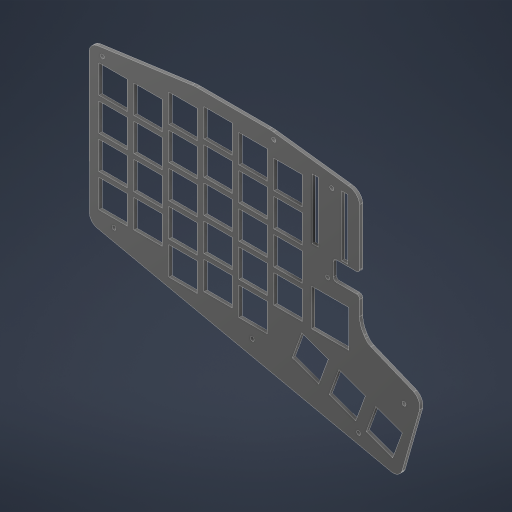
# Autodesk Inventor part: Top plate Right
Saved by Autodesk Inventor 2024.3 (Build 283343000, 343)
## iProperties
Created: 2024-12-13
Part Number: Top plate Right
Material: ABS Plastic
Document SubType Name: Modeling
Designer: micha
Density: 1.06 g/cm^3
Appearance: Smooth - Black
Author: micha
Autodesk Inventor part; units mm, degrees
ref_plane "YZ Plane" through (0, 0, 0) normal (1, 0, 0) x (0, 1, 0)
ref_plane "XZ Plane" through (0, 0, 0) normal (0, 1, 0) x (-1, 0, 0)
ref_plane "Work Plane1" through (0, 0, 0) normal (0, 0, 1) x (1, 0, 0)
sketch "Sketch1" plane through (0, 0, 0) normal (0, 0, 1) x (1, 0, 0)
  arc A0 (218.5045, -64.8588) -> (212.539, -59.4694) centre (212.5401, -65.4644) ccw projected
  line L0 (174.0364, -54.7609) -> (212.539, -59.4694) projected
  arc A1 (174.0364, -54.7609) -> (171.7239, -54.62) centre (171.7239, -73.6702) ccw projected
  line L1 (134.8832, -54.62) -> (171.7239, -54.62) projected
  arc A2 (134.8832, -54.62) -> (132.2802, -54.7987) centre (134.8832, -73.6711) ccw projected
  line L2 (83.5422, -61.5211) -> (132.2802, -54.7987) projected
  arc A3 (83.5422, -61.5211) -> (79.23, -66.4736) centre (84.23, -66.4736) ccw projected
  line L3 (79.4773, -138.0224) -> (79.23, -66.4736) projected
  arc A4 (79.4773, -138.0224) -> (82.9877, -142.7953) centre (84.4773, -138.0223) ccw projected
  line L4 (234.3607, -175.7237) -> (82.9877, -142.7953) projected
  arc A5 (234.3607, -175.7237) -> (240.2338, -172.8773) centre (235.7454, -171.0986) ccw projected
  line L5 (249.3284, -140.9769) -> (240.2338, -172.8773) projected
  arc A6 (249.3284, -140.9769) -> (246.2558, -134.3964) centre (243.557, -139.6641) ccw projected
  line L6 (224.2532, -125.4096) -> (246.2558, -134.3964) projected
  arc A7 (221.4228, -123.1302) -> (224.2532, -125.4096) centre (226.6543, -119.531) ccw projected
  line L7 (220.6818, -122.0531) -> (221.4228, -123.1302) projected
  arc A8 (218.4447, -114.8395) -> (220.6818, -122.0531) centre (231.1445, -114.8548) ccw projected
  line L8 (218.5045, -64.8588) -> (218.4447, -114.8395) projected
  circle A9 centre (163.195, -152.4) radius 1.05 projected
  circle A10 centre (92.075, -138.43) radius 1.05 projected
  circle A11 centre (86.11, -127.04) radius 0.8509 projected
  circle A12 centre (91.61, -127.04) radius 1.7145 projected
  circle A13 centre (97.11, -127.04) radius 0.8509 projected
  circle A14 centre (104.11, -127.04) radius 0.8509 projected
  circle A15 centre (122.11, -139.04) radius 0.8509 projected
  circle A16 centre (122.61, -135.29) radius 1.5 projected
  circle A17 centre (109.61, -127.04) radius 1.7145 projected
  circle A18 centre (115.11, -127.04) radius 0.8509 projected
  circle A19 centre (86.61, -123.29) radius 1.5 projected
  circle A20 centre (91.61, -121.09) radius 1.5 projected
  circle A21 centre (96.61, -123.29) radius 1.5 projected
  circle A22 centre (104.61, -123.29) radius 1.5 projected
  circle A23 centre (109.61, -121.09) radius 1.5 projected
  circle A24 centre (114.61, -123.29) radius 1.5 projected
  circle A25 centre (122.11, -122.04) radius 0.8509 projected
  circle A26 centre (122.61, -118.29) radius 1.5 projected
  circle A27 centre (127.61, -139.04) radius 1.7145 projected
  circle A28 centre (133.11, -139.04) radius 0.8509 projected
  circle A29 centre (132.61, -135.29) radius 1.5 projected
  circle A30 centre (140.11, -136.54) radius 0.8509 projected
  circle A31 centre (127.61, -133.09) radius 1.5 projected
  circle A32 centre (140.61, -132.79) radius 1.5 projected
  circle A33 centre (145.61, -136.54) radius 1.7145 projected
  circle A34 centre (151.11, -136.54) radius 0.8509 projected
  circle A35 centre (158.11, -139.04) radius 0.8509 projected
  circle A36 centre (163.61, -139.04) radius 1.7145 projected
  circle A37 centre (158.61, -135.29) radius 1.5 projected
  circle A38 centre (145.61, -130.59) radius 1.5 projected
  circle A39 centre (150.61, -132.79) radius 1.5 projected
  circle A40 centre (163.61, -133.09) radius 1.5 projected
  circle A41 centre (127.61, -122.04) radius 1.7145 projected
  circle A42 centre (133.11, -122.04) radius 0.8509 projected
  circle A43 centre (140.11, -119.54) radius 0.8509 projected
  circle A44 centre (127.61, -116.09) radius 1.5 projected
  circle A45 centre (132.61, -118.29) radius 1.5 projected
  circle A46 centre (140.61, -115.79) radius 1.5 projected
  circle A47 centre (145.61, -119.54) radius 1.7145 projected
  circle A48 centre (151.11, -119.54) radius 0.8509 projected
  circle A49 centre (158.11, -122.04) radius 0.8509 projected
  circle A50 centre (163.61, -122.04) radius 1.7145 projected
  circle A51 centre (145.61, -113.59) radius 1.5 projected
  circle A52 centre (150.61, -115.79) radius 1.5 projected
  circle A53 centre (158.61, -118.29) radius 1.5 projected
  circle A54 centre (163.61, -116.09) radius 1.5 projected
  circle A55 centre (198.2508, -148.0493) radius 0.8509 projected
  circle A56 centre (187.9141, -144.2871) radius 0.8509 projected
  circle A57 centre (193.0824, -146.1682) radius 1.7145 projected
  circle A58 centre (189.6666, -140.9342) radius 1.5 projected
  circle A59 centre (199.0635, -144.3544) radius 1.5 projected
  circle A60 centre (195.1175, -140.577) radius 1.5 projected
  circle A61 centre (217.8966, -166.9609) radius 1.05 projected
  circle A62 centre (217.2795, -154.9752) radius 0.8509 projected
  circle A63 centre (236.3083, -161.9011) radius 0.8509 projected
  circle A64 centre (225.9717, -158.1389) radius 0.8509 projected
  circle A65 centre (231.14, -160.02) radius 1.7145 projected
  circle A66 centre (227.7241, -154.7861) radius 1.5 projected
  circle A67 centre (237.121, -158.2063) radius 1.5 projected
  circle A68 centre (233.175, -154.4288) radius 1.5 projected
  circle A69 centre (206.9429, -151.213) radius 0.8509 projected
  circle A70 centre (212.1112, -153.0941) radius 1.7145 projected
  circle A71 centre (208.6953, -147.8601) radius 1.5 projected
  circle A72 centre (218.0923, -151.2803) radius 1.5 projected
  circle A73 centre (214.1462, -147.5029) radius 1.5 projected
  circle A74 centre (241.3, -142.24) radius 1.05 projected
  circle A75 centre (169.11, -139.04) radius 0.8509 projected
  circle A76 centre (168.61, -135.29) radius 1.5 projected
  circle A77 centre (201.8629, -128.353) radius 0.8509 projected
  circle A78 centre (169.11, -122.04) radius 0.8509 projected
  circle A79 centre (176.11, -124.54) radius 0.8509 projected
  circle A80 centre (181.61, -124.54) radius 1.7145 projected
  circle A81 centre (176.61, -120.79) radius 1.5 projected
  circle A82 centre (168.61, -118.29) radius 1.5 projected
  circle A83 centre (181.61, -118.59) radius 1.5 projected
  circle A84 centre (187.11, -124.54) radius 0.8509 projected
  circle A85 centre (186.61, -120.79) radius 1.5 projected
  circle A86 centre (194.5006, -125.0592) radius 0.4 projected
  circle A87 centre (194.5006, -123.0592) radius 0.381 projected
  circle A88 centre (194.5006, -121.0592) radius 0.381 projected
  circle A89 centre (201.3506, -114.2092) radius 0.4 projected
  circle A90 centre (220.8917, -135.2789) radius 0.8509 projected
  circle A91 centre (207.0312, -130.2341) radius 1.7145 projected
  circle A92 centre (212.1995, -132.1152) radius 0.8509 projected
  circle A93 centre (222.6441, -131.9261) radius 1.5 projected
  circle A94 centre (213.0123, -128.4203) radius 1.5 projected
  circle A95 centre (226.06, -137.16) radius 1.7145 projected
  circle A96 centre (231.2283, -139.0411) radius 0.8509 projected
  circle A97 centre (232.041, -135.3463) radius 1.5 projected
  circle A98 centre (228.095, -131.5688) radius 1.5 projected
  circle A99 centre (203.6153, -125.0001) radius 1.5 projected
  circle A100 centre (209.0662, -124.6429) radius 1.5 projected
  circle A101 centre (203.3506, -114.2092) radius 0.4 projected
  circle A102 centre (205.3506, -114.2092) radius 0.4 projected
  circle A103 centre (86.11, -110.04) radius 0.8509 projected
  circle A104 centre (91.61, -110.04) radius 1.7145 projected
  circle A105 centre (86.61, -106.29) radius 1.5 projected
  circle A106 centre (97.11, -110.04) radius 0.8509 projected
  circle A107 centre (104.11, -110.04) radius 0.8509 projected
  circle A108 centre (96.61, -106.29) radius 1.5 projected
  circle A109 centre (104.61, -106.29) radius 1.5 projected
  circle A110 centre (91.61, -104.09) radius 1.5 projected
  circle A111 centre (109.61, -110.04) radius 1.7145 projected
  circle A112 centre (115.11, -110.04) radius 0.8509 projected
  circle A113 centre (114.61, -106.29) radius 1.5 projected
  circle A114 centre (109.61, -104.09) radius 1.5 projected
  circle A115 centre (122.11, -105.04) radius 0.8509 projected
  circle A116 centre (122.61, -101.29) radius 1.5 projected
  circle A117 centre (86.11, -93.04) radius 0.8509 projected
  circle A118 centre (91.61, -93.04) radius 1.7145 projected
  circle A119 centre (97.11, -93.04) radius 0.8509 projected
  circle A120 centre (104.11, -93.04) radius 0.8509 projected
  circle A121 centre (86.61, -89.29) radius 1.5 projected
  circle A122 centre (91.61, -87.09) radius 1.5 projected
  circle A123 centre (96.61, -89.29) radius 1.5 projected
  circle A124 centre (104.61, -89.29) radius 1.5 projected
  circle A125 centre (109.61, -93.04) radius 1.7145 projected
  circle A126 centre (115.11, -93.04) radius 0.8509 projected
  circle A127 centre (109.61, -87.09) radius 1.5 projected
  circle A128 centre (114.61, -89.29) radius 1.5 projected
  circle A129 centre (122.11, -88.04) radius 0.8509 projected
  circle A130 centre (127.61, -105.04) radius 1.7145 projected
  circle A131 centre (133.11, -105.04) radius 0.8509 projected
  circle A132 centre (127.61, -99.09) radius 1.5 projected
  circle A133 centre (132.61, -101.29) radius 1.5 projected
  circle A134 centre (140.11, -102.54) radius 0.8509 projected
  circle A135 centre (140.61, -98.79) radius 1.5 projected
  circle A136 centre (145.61, -102.54) radius 1.7145 projected
  circle A137 centre (151.11, -102.54) radius 0.8509 projected
  circle A138 centre (150.61, -98.79) radius 1.5 projected
  circle A139 centre (158.11, -105.04) radius 0.8509 projected
  circle A140 centre (163.61, -105.04) radius 1.7145 projected
  circle A141 centre (158.61, -101.29) radius 1.5 projected
  circle A142 centre (163.61, -99.09) radius 1.5 projected
  circle A143 centre (127.61, -88.04) radius 1.7145 projected
  circle A144 centre (133.11, -88.04) radius 0.8509 projected
  circle A145 centre (140.11, -85.54) radius 0.8509 projected
  circle A146 centre (145.61, -96.59) radius 1.5 projected
  circle A147 centre (145.61, -85.54) radius 1.7145 projected
  circle A148 centre (151.11, -85.54) radius 0.8509 projected
  circle A149 centre (158.11, -88.04) radius 0.8509 projected
  circle A150 centre (163.61, -88.04) radius 1.7145 projected
  circle A151 centre (86.11, -76.04) radius 0.8509 projected
  circle A152 centre (91.61, -76.04) radius 1.7145 projected
  circle A153 centre (86.61, -72.29) radius 1.5 projected
  circle A154 centre (97.11, -76.04) radius 0.8509 projected
  circle A155 centre (104.11, -76.04) radius 0.8509 projected
  circle A156 centre (96.61, -72.29) radius 1.5 projected
  circle A157 centre (104.61, -72.29) radius 1.5 projected
  circle A158 centre (122.61, -84.29) radius 1.5 projected
  circle A159 centre (109.61, -76.04) radius 1.7145 projected
  circle A160 centre (115.11, -76.04) radius 0.8509 projected
  circle A161 centre (114.61, -72.29) radius 1.5 projected
  circle A162 centre (122.11, -71.04) radius 0.8509 projected
  circle A163 centre (91.61, -70.09) radius 1.5 projected
  circle A164 centre (86.1194, -65.1034) radius 1.05 projected
  circle A165 centre (109.61, -70.09) radius 1.5 projected
  circle A166 centre (122.61, -67.29) radius 1.5 projected
  circle A167 centre (127.61, -82.09) radius 1.5 projected
  circle A168 centre (132.61, -84.29) radius 1.5 projected
  circle A169 centre (140.61, -81.79) radius 1.5 projected
  circle A170 centre (127.61, -71.04) radius 1.7145 projected
  circle A171 centre (133.11, -71.04) radius 0.8509 projected
  circle A172 centre (150.61, -81.79) radius 1.5 projected
  circle A173 centre (145.61, -79.59) radius 1.5 projected
  circle A174 centre (158.61, -84.29) radius 1.5 projected
  circle A175 centre (163.61, -82.09) radius 1.5 projected
  circle A176 centre (158.11, -71.04) radius 0.8509 projected
  circle A177 centre (163.61, -71.04) radius 1.7145 projected
  circle A178 centre (127.61, -65.09) radius 1.5 projected
  circle A179 centre (132.61, -67.29) radius 1.5 projected
  circle A180 centre (140.11, -68.54) radius 0.8509 projected
  circle A181 centre (140.61, -64.79) radius 1.5 projected
  circle A182 centre (145.61, -68.54) radius 1.7145 projected
  circle A183 centre (151.11, -68.54) radius 0.8509 projected
  circle A184 centre (150.61, -64.79) radius 1.5 projected
  circle A185 centre (158.61, -67.29) radius 1.5 projected
  circle A186 centre (163.61, -65.09) radius 1.5 projected
  circle A187 centre (145.61, -62.59) radius 1.5 projected
  circle A188 centre (176.11, -107.54) radius 0.8509 projected
  circle A189 centre (181.61, -107.54) radius 1.7145 projected
  circle A190 centre (169.11, -105.04) radius 0.8509 projected
  circle A191 centre (168.61, -101.29) radius 1.5 projected
  circle A192 centre (176.61, -103.79) radius 1.5 projected
  circle A193 centre (181.61, -101.59) radius 1.5 projected
  circle A194 centre (187.11, -107.54) radius 0.8509 projected
  circle A195 centre (202.0465, -105.6044) radius 1.05 projected
  circle A196 centre (186.61, -103.79) radius 1.5 projected
  circle A197 centre (169.11, -88.04) radius 0.8509 projected
  circle A198 centre (176.11, -90.54) radius 0.8509 projected
  circle A199 centre (181.61, -90.54) radius 1.7145 projected
  circle A200 centre (176.61, -86.79) radius 1.5 projected
  circle A201 centre (195.58, -92.9563) radius 0.5461 projected
  circle A202 centre (187.11, -90.54) radius 0.8509 projected
  circle A203 centre (186.61, -86.79) radius 1.5 projected
  circle A204 centre (195.58, -90.4163) radius 0.5461 projected
  circle A205 centre (195.58, -87.8763) radius 0.5461 projected
  circle A206 centre (195.58, -85.3363) radius 0.5461 projected
  arc A207 (207.5558, -103.5294) -> (207.5558, -104.4294) centre (207.5558, -103.9794) ccw projected
  line L9 (207.5558, -103.5294) -> (208.1558, -103.5294) projected
  arc A208 (208.1558, -104.4294) -> (208.1558, -103.5294) centre (208.1558, -103.9794) ccw projected
  line L10 (208.1558, -104.4294) -> (207.5558, -104.4294) projected
  arc A209 (211.5558, -103.5294) -> (211.5558, -104.4294) centre (211.5558, -103.9794) ccw projected
  line L11 (211.5558, -103.5294) -> (212.1558, -103.5294) projected
  arc A210 (212.1558, -104.4294) -> (212.1558, -103.5294) centre (212.1558, -103.9794) ccw projected
  line L12 (212.1558, -104.4294) -> (211.5558, -104.4294) projected
  arc A211 (206.4558, -101.2294) -> (206.4558, -102.1294) centre (206.4558, -101.6794) ccw projected
  line L13 (206.4558, -101.2294) -> (207.0558, -101.2294) projected
  arc A212 (207.0558, -102.1294) -> (207.0558, -101.2294) centre (207.0558, -101.6794) ccw projected
  line L14 (207.0558, -102.1294) -> (206.4558, -102.1294) projected
  arc A213 (206.4558, -98.9294) -> (206.4558, -99.8294) centre (206.4558, -99.3794) ccw projected
  line L15 (206.4558, -98.9294) -> (207.0558, -98.9294) projected
  arc A214 (207.0558, -99.8294) -> (207.0558, -98.9294) centre (207.0558, -99.3794) ccw projected
  line L16 (207.0558, -99.8294) -> (206.4558, -99.8294) projected
  circle A215 centre (209.4558, -101.6794) radius 0.75 projected
  circle A216 centre (209.4558, -99.3794) radius 0.75 projected
  arc A217 (214.5558, -103.5294) -> (214.5558, -104.4294) centre (214.5558, -103.9794) ccw projected
  line L17 (214.5558, -103.5294) -> (215.1558, -103.5294) projected
  arc A218 (215.1558, -104.4294) -> (215.1558, -103.5294) centre (215.1558, -103.9794) ccw projected
  line L18 (215.1558, -104.4294) -> (214.5558, -104.4294) projected
  circle A219 centre (216.4558, -101.6794) radius 0.75 projected
  circle A220 centre (216.4558, -99.3794) radius 0.75 projected
  arc A221 (207.5558, -96.6294) -> (207.5558, -97.5294) centre (207.5558, -97.0794) ccw projected
  line L19 (207.5558, -96.6294) -> (208.1558, -96.6294) projected
  arc A222 (208.1558, -97.5294) -> (208.1558, -96.6294) centre (208.1558, -97.0794) ccw projected
  line L20 (208.1558, -97.5294) -> (207.5558, -97.5294) projected
  arc A223 (211.5558, -96.6294) -> (211.5558, -97.5294) centre (211.5558, -97.0794) ccw projected
  line L21 (211.5558, -96.6294) -> (212.1558, -96.6294) projected
  arc A224 (212.1558, -97.5294) -> (212.1558, -96.6294) centre (212.1558, -97.0794) ccw projected
  line L22 (212.1558, -97.5294) -> (211.5558, -97.5294) projected
  circle A225 centre (210.82, -92.9563) radius 0.5461 projected
  arc A226 (214.5558, -96.6294) -> (214.5558, -97.5294) centre (214.5558, -97.0794) ccw projected
  line L23 (214.5558, -96.6294) -> (215.1558, -96.6294) projected
  arc A227 (215.1558, -97.5294) -> (215.1558, -96.6294) centre (215.1558, -97.0794) ccw projected
  line L24 (215.1558, -97.5294) -> (214.5558, -97.5294) projected
  circle A228 centre (210.82, -90.4163) radius 0.5461 projected
  circle A229 centre (210.82, -87.8763) radius 0.5461 projected
  circle A230 centre (210.82, -85.3363) radius 0.5461 projected
  circle A231 centre (168.61, -84.29) radius 1.5 projected
  circle A232 centre (181.61, -84.59) radius 1.5 projected
  circle A233 centre (169.11, -71.04) radius 0.8509 projected
  circle A234 centre (176.11, -73.54) radius 0.8509 projected
  circle A235 centre (181.61, -73.54) radius 1.7145 projected
  circle A236 centre (195.58, -82.7963) radius 0.5461 projected
  circle A237 centre (195.58, -80.2563) radius 0.5461 projected
  circle A238 centre (187.11, -73.54) radius 0.8509 projected
  circle A239 centre (195.58, -77.7163) radius 0.5461 projected
  circle A240 centre (195.58, -75.1763) radius 0.5461 projected
  circle A241 centre (199.5, -77.7363) radius 0.2 projected
  circle A242 centre (199.45, -75.2863) radius 0.2 projected
  circle A243 centre (195.58, -72.6363) radius 0.5461 projected
  circle A244 centre (199.45, -72.6363) radius 0.2 projected
  circle A245 centre (168.61, -67.29) radius 1.5 projected
  circle A246 centre (176.61, -69.79) radius 1.5 projected
  circle A247 centre (181.61, -67.59) radius 1.5 projected
  circle A248 centre (174.3426, -58.0743) radius 1.05 projected
  circle A249 centre (186.61, -69.79) radius 1.5 projected
  circle A250 centre (195.58, -70.0963) radius 0.5461 projected
  circle A251 centre (195.58, -67.5563) radius 0.5461 projected
  circle A252 centre (199.4864, -69.9863) radius 0.2 projected
  circle A253 centre (195.58, -65.0163) radius 0.5461 projected
  circle A254 centre (210.82, -82.7963) radius 0.5461 projected
  circle A255 centre (210.82, -80.2563) radius 0.5461 projected
  circle A256 centre (206.55, -77.7863) radius 0.2 projected
  circle A257 centre (206.55, -75.2363) radius 0.2 projected
  circle A258 centre (210.82, -77.7163) radius 0.5461 projected
  circle A259 centre (210.82, -75.1763) radius 0.5461 projected
  circle A260 centre (206.55, -72.6363) radius 0.2 projected
  circle A261 centre (210.82, -72.6363) radius 0.5461 projected
  circle A262 centre (206.55, -70.1863) radius 0.2 projected
  circle A263 centre (210.82, -70.0963) radius 0.5461 projected
  circle A264 centre (210.82, -67.5563) radius 0.5461 projected
  circle A265 centre (204.2038, -64.7368) radius 1.05 projected
  circle A266 centre (210.82, -65.0163) radius 0.5461 projected
  line L25 (84.371, -83.279) -> (98.849, -83.279)
  line L26 (98.849, -83.279) -> (98.849, -68.801)
  line L27 (98.849, -68.801) -> (84.371, -68.801)
  line L28 (84.371, -68.801) -> (84.371, -83.279)
  line L29 (84.371, -83.279) -> (98.849, -68.801) construction
  line L30 (98.849, -83.279) -> (84.371, -68.801) construction
  line L31 (91.61, -76.04) -> (94.8856, -76.04) construction
  line L32 (91.61, -76.04) -> (91.61, -78.956) construction
  line L33 (102.371, -68.801) -> (116.849, -68.801)
  line L34 (116.849, -68.801) -> (116.849, -83.279)
  line L35 (116.849, -83.279) -> (102.371, -83.279)
  line L36 (102.371, -83.279) -> (102.371, -68.801)
  line L37 (102.371, -68.801) -> (116.849, -83.279) construction
  line L38 (116.849, -68.801) -> (102.371, -83.279) construction
  line L39 (120.371, -78.279) -> (134.849, -78.279)
  line L40 (134.849, -78.279) -> (134.849, -63.801)
  line L41 (134.849, -63.801) -> (120.371, -63.801)
  line L42 (120.371, -63.801) -> (120.371, -78.279)
  line L43 (120.371, -78.279) -> (134.849, -63.801) construction
  line L44 (134.849, -78.279) -> (120.371, -63.801) construction
  line L45 (138.371, -75.779) -> (152.849, -75.779)
  line L46 (152.849, -75.779) -> (152.849, -61.301)
  line L47 (152.849, -61.301) -> (138.371, -61.301)
  line L48 (138.371, -61.301) -> (138.371, -75.779)
  line L49 (138.371, -75.779) -> (152.849, -61.301) construction
  line L50 (152.849, -75.779) -> (138.371, -61.301) construction
  line L51 (156.371, -78.279) -> (170.849, -78.279)
  line L52 (170.849, -78.279) -> (170.849, -63.801)
  line L53 (170.849, -63.801) -> (156.371, -63.801)
  line L54 (156.371, -63.801) -> (156.371, -78.279)
  line L55 (156.371, -78.279) -> (170.849, -63.801) construction
  line L56 (170.849, -78.279) -> (156.371, -63.801) construction
  line L57 (174.371, -80.779) -> (188.849, -80.779)
  line L58 (188.849, -80.779) -> (188.849, -66.301)
  line L59 (188.849, -66.301) -> (174.371, -66.301)
  line L60 (174.371, -66.301) -> (174.371, -80.779)
  line L61 (174.371, -80.779) -> (188.849, -66.301) construction
  line L62 (188.849, -80.779) -> (174.371, -66.301) construction
  line L63 (84.371, -100.279) -> (98.849, -100.279)
  line L64 (98.849, -100.279) -> (98.849, -85.801)
  line L65 (98.849, -85.801) -> (84.371, -85.801)
  line L66 (84.371, -85.801) -> (84.371, -100.279)
  line L67 (84.371, -100.279) -> (98.849, -85.801) construction
  line L68 (98.849, -100.279) -> (84.371, -85.801) construction
  line L69 (102.371, -100.279) -> (116.849, -100.279)
  line L70 (116.849, -100.279) -> (116.849, -85.801)
  line L71 (116.849, -85.801) -> (102.371, -85.801)
  line L72 (102.371, -85.801) -> (102.371, -100.279)
  line L73 (102.371, -100.279) -> (116.849, -85.801) construction
  line L74 (116.849, -100.279) -> (102.371, -85.801) construction
  line L75 (120.371, -95.279) -> (134.849, -95.279)
  line L76 (134.849, -95.279) -> (134.849, -80.801)
  line L77 (134.849, -80.801) -> (120.371, -80.801)
  line L78 (120.371, -80.801) -> (120.371, -95.279)
  line L79 (120.371, -95.279) -> (134.849, -80.801) construction
  line L80 (134.849, -95.279) -> (120.371, -80.801) construction
  line L81 (138.371, -92.779) -> (152.849, -92.779)
  line L82 (152.849, -92.779) -> (152.849, -78.301)
  line L83 (152.849, -78.301) -> (138.371, -78.301)
  line L84 (138.371, -78.301) -> (138.371, -92.779)
  line L85 (138.371, -92.779) -> (152.849, -78.301) construction
  line L86 (152.849, -92.779) -> (138.371, -78.301) construction
  line L87 (156.371, -95.279) -> (170.849, -95.279)
  line L88 (170.849, -95.279) -> (170.849, -80.801)
  line L89 (170.849, -80.801) -> (156.371, -80.801)
  line L90 (156.371, -80.801) -> (156.371, -95.279)
  line L91 (156.371, -95.279) -> (170.849, -80.801) construction
  line L92 (170.849, -95.279) -> (156.371, -80.801) construction
  line L93 (174.371, -97.779) -> (188.849, -97.779)
  line L94 (188.849, -97.779) -> (188.849, -83.301)
  line L95 (188.849, -83.301) -> (174.371, -83.301)
  line L96 (174.371, -83.301) -> (174.371, -97.779)
  line L97 (174.371, -97.779) -> (188.849, -83.301) construction
  line L98 (188.849, -97.779) -> (174.371, -83.301) construction
  line L99 (174.371, -114.779) -> (188.849, -114.779)
  line L100 (188.849, -114.779) -> (188.849, -100.301)
  line L101 (188.849, -100.301) -> (174.371, -100.301)
  line L102 (174.371, -100.301) -> (174.371, -114.779)
  line L103 (174.371, -114.779) -> (188.849, -100.301) construction
  line L104 (188.849, -114.779) -> (174.371, -100.301) construction
  line L105 (156.371, -112.279) -> (170.849, -112.279)
  line L106 (170.849, -112.279) -> (170.849, -97.801)
  line L107 (170.849, -97.801) -> (156.371, -97.801)
  line L108 (156.371, -97.801) -> (156.371, -112.279)
  line L109 (156.371, -112.279) -> (170.849, -97.801) construction
  line L110 (170.849, -112.279) -> (156.371, -97.801) construction
  line L111 (138.371, -109.779) -> (152.849, -109.779)
  line L112 (152.849, -109.779) -> (152.849, -95.301)
  line L113 (152.849, -95.301) -> (138.371, -95.301)
  line L114 (138.371, -95.301) -> (138.371, -109.779)
  line L115 (138.371, -109.779) -> (152.849, -95.301) construction
  line L116 (152.849, -109.779) -> (138.371, -95.301) construction
  line L117 (120.371, -112.279) -> (134.849, -112.279)
  line L118 (134.849, -112.279) -> (134.849, -97.801)
  line L119 (134.849, -97.801) -> (120.371, -97.801)
  line L120 (120.371, -97.801) -> (120.371, -112.279)
  line L121 (120.371, -112.279) -> (134.849, -97.801) construction
  line L122 (134.849, -112.279) -> (120.371, -97.801) construction
  line L123 (102.371, -117.279) -> (116.849, -117.279)
  line L124 (116.849, -117.279) -> (116.849, -102.801)
  line L125 (116.849, -102.801) -> (102.371, -102.801)
  line L126 (102.371, -102.801) -> (102.371, -117.279)
  line L127 (102.371, -117.279) -> (116.849, -102.801) construction
  line L128 (116.849, -117.279) -> (102.371, -102.801) construction
  line L129 (84.371, -117.279) -> (98.849, -117.279)
  line L130 (98.849, -117.279) -> (98.849, -102.801)
  line L131 (98.849, -102.801) -> (84.371, -102.801)
  line L132 (84.371, -102.801) -> (84.371, -117.279)
  line L133 (84.371, -117.279) -> (98.849, -102.801) construction
  line L134 (98.849, -117.279) -> (84.371, -102.801) construction
  line L135 (84.371, -134.279) -> (98.849, -134.279)
  line L136 (98.849, -134.279) -> (98.849, -119.801)
  line L137 (98.849, -119.801) -> (84.371, -119.801)
  line L138 (84.371, -119.801) -> (84.371, -134.279)
  line L139 (84.371, -134.279) -> (98.849, -119.801) construction
  line L140 (98.849, -134.279) -> (84.371, -119.801) construction
  line L141 (102.371, -134.279) -> (116.849, -134.279)
  line L142 (116.849, -134.279) -> (116.849, -119.801)
  line L143 (116.849, -119.801) -> (102.371, -119.801)
  line L144 (102.371, -119.801) -> (102.371, -134.279)
  line L145 (102.371, -134.279) -> (116.849, -119.801) construction
  line L146 (116.849, -134.279) -> (102.371, -119.801) construction
  line L147 (120.371, -129.279) -> (134.849, -129.279)
  line L148 (134.849, -129.279) -> (134.849, -114.801)
  line L149 (134.849, -114.801) -> (120.371, -114.801)
  line L150 (120.371, -114.801) -> (120.371, -129.279)
  line L151 (120.371, -129.279) -> (134.849, -114.801) construction
  line L152 (134.849, -129.279) -> (120.371, -114.801) construction
  line L153 (138.371, -126.779) -> (152.849, -126.779)
  line L154 (152.849, -126.779) -> (152.849, -112.301)
  line L155 (152.849, -112.301) -> (138.371, -112.301)
  line L156 (138.371, -112.301) -> (138.371, -126.779)
  line L157 (138.371, -126.779) -> (152.849, -112.301) construction
  line L158 (152.849, -126.779) -> (138.371, -112.301) construction
  line L159 (156.371, -129.279) -> (170.849, -129.279)
  line L160 (170.849, -129.279) -> (170.849, -114.801)
  line L161 (170.849, -114.801) -> (156.371, -114.801)
  line L162 (156.371, -114.801) -> (156.371, -129.279)
  line L163 (156.371, -129.279) -> (170.849, -114.801) construction
  line L164 (170.849, -129.279) -> (156.371, -114.801) construction
  line L165 (174.371, -131.779) -> (188.849, -131.779)
  line L166 (188.849, -131.779) -> (188.849, -117.301)
  line L167 (188.849, -117.301) -> (174.371, -117.301)
  line L168 (174.371, -117.301) -> (174.371, -131.779)
  line L169 (174.371, -131.779) -> (188.849, -117.301) construction
  line L170 (188.849, -131.779) -> (174.371, -117.301) construction
  line L171 (156.371, -146.279) -> (170.849, -146.279)
  line L172 (170.849, -146.279) -> (170.849, -131.801)
  line L173 (170.849, -131.801) -> (156.371, -131.801)
  line L174 (156.371, -131.801) -> (156.371, -146.279)
  line L175 (156.371, -146.279) -> (170.849, -131.801) construction
  line L176 (170.849, -146.279) -> (156.371, -131.801) construction
  line L177 (138.371, -143.779) -> (152.849, -143.779)
  line L178 (152.849, -143.779) -> (152.849, -129.301)
  line L179 (152.849, -129.301) -> (138.371, -129.301)
  line L180 (138.371, -129.301) -> (138.371, -143.779)
  line L181 (138.371, -143.779) -> (152.849, -129.301) construction
  line L182 (152.849, -143.779) -> (138.371, -129.301) construction
  line L183 (120.371, -146.279) -> (134.849, -146.279)
  line L184 (134.849, -146.279) -> (134.849, -131.801)
  line L185 (134.849, -131.801) -> (120.371, -131.801)
  line L186 (120.371, -131.801) -> (120.371, -146.279)
  line L187 (120.371, -146.279) -> (134.849, -131.801) construction
  line L188 (134.849, -146.279) -> (120.371, -131.801) construction
  line L189 (187.9141, -144.2871) -> (198.2508, -148.0493) construction
  line L190 (193.0824, -146.1682) -> (195.1175, -140.577) construction
  line L191 (202.3608, -141.8416) -> (197.409, -155.4465)
  line L192 (197.409, -155.4465) -> (183.8041, -150.4947)
  line L193 (183.8041, -150.4947) -> (188.7559, -136.8899)
  line L194 (188.7559, -136.8899) -> (202.3608, -141.8416)
  line L195 (221.3895, -148.7675) -> (216.4378, -162.3724)
  line L196 (216.4378, -162.3724) -> (202.8329, -157.4206)
  line L197 (202.8329, -157.4206) -> (207.7847, -143.8158)
  line L198 (207.7847, -143.8158) -> (221.3895, -148.7675)
  line L199 (240.4183, -155.6934) -> (235.4666, -169.2983)
  line L200 (235.4666, -169.2983) -> (221.8617, -164.3466)
  line L201 (221.8617, -164.3466) -> (226.8134, -150.7417)
  line L202 (226.8134, -150.7417) -> (240.4183, -155.6934)
  line L203 (235.3383, -132.8334) -> (230.3866, -146.4383)
  line L204 (230.3866, -146.4383) -> (216.7817, -141.4866)
  line L205 (216.7817, -141.4866) -> (221.7334, -127.8817)
  line L206 (221.7334, -127.8817) -> (235.3383, -132.8334)
  line L207 (216.3095, -125.9075) -> (211.3578, -139.5124)
  line L208 (211.3578, -139.5124) -> (197.7529, -134.5606)
  line L209 (197.7529, -134.5606) -> (202.7047, -120.9558)
  line L210 (202.7047, -120.9558) -> (216.3095, -125.9075)
  line L211 (194.5006, -123.0592) -> (203.3506, -123.0592) construction
  line L212 (203.3506, -123.0592) -> (203.3506, -114.2092) construction
  line L213 (194.5006, -121.0592) -> (194.5006, -123.0592) construction
  line L214 (212.8756, -132.5842) -> (193.8256, -132.5842)
  line L215 (193.8256, -132.5842) -> (193.8256, -113.5342)
  line L216 (193.8256, -113.5342) -> (212.8756, -113.5342)
  line L217 (212.8756, -113.5342) -> (212.8756, -132.5842)
  line L218 (212.8756, -132.5842) -> (193.8256, -113.5342) construction
  line L219 (193.8256, -132.5842) -> (212.8756, -113.5342) construction
  line L220 (206.4558, -99.3794) -> (206.4558, -101.6794) construction
  line L221 (207.5558, -103.9794) -> (215.1558, -103.9794) construction
  line L222 (215.1558, -97.0794) -> (207.5558, -97.0794) construction
  line L223 (193.9925, -63.4288) -> (197.1675, -63.4288)
  line L224 (197.1675, -63.4288) -> (197.1675, -94.5438)
  line L225 (197.1675, -94.5438) -> (193.9925, -94.5438)
  line L226 (193.9925, -94.5438) -> (193.9925, -63.4288)
  line L227 (209.2325, -63.4288) -> (212.4075, -63.4288)
  line L228 (212.4075, -63.4288) -> (212.4075, -94.5438)
  line L229 (212.4075, -94.5438) -> (209.2325, -94.5438)
  line L230 (209.2325, -94.5438) -> (209.2325, -63.4288)
  line L231 (218.4558, -105.5669) -> (204.8683, -105.5669)
  line L232 (218.4679, -95.4919) -> (204.8683, -95.4919)
  line L233 (204.8683, -95.4919) -> (204.8683, -105.5669)
  point P0 (0, 0)
  point P1 (193.0824, -146.1682)
  point P2 (208.7862, -123.1693)
  point P3 (210.228, -123.694)
  dimension "d2" = 14.478
  dimension "d3" = 14.478
  dimension "d4" = 14.478
  dimension "d5" = 14.478
  dimension "d6" = 14.478
  dimension "d7" = 14.478
  dimension "d8" = 14.478
  dimension "d9" = 14.478
  dimension "d10" = 14.478
  dimension "d11" = 14.478
  dimension "d12" = 14.478
  dimension "d13" = 14.478
  dimension "d14" = 14.478
  dimension "d15" = 14.478
  dimension "d16" = 14.478
  dimension "d17" = 14.478
  dimension "d18" = 14.478
  dimension "d19" = 14.478
  dimension "d20" = 14.478
  dimension "d21" = 14.478
  dimension "d22" = 14.478
  dimension "d23" = 14.478
  dimension "d24" = 14.478
  dimension "d25" = 14.478
  dimension "d26" = 14.478
  dimension "d27" = 14.478
  dimension "d28" = 14.478
  dimension "d29" = 14.478
  dimension "d30" = 14.478
  dimension "d31" = 14.478
  dimension "d32" = 14.478
  dimension "d33" = 14.478
  dimension "d34" = 14.478
  dimension "d35" = 14.478
  dimension "d36" = 14.478
  dimension "d37" = 14.478
  dimension "d38" = 14.478
  dimension "d39" = 14.478
  dimension "d40" = 14.478
  dimension "d41" = 14.478
  dimension "d42" = 14.478
  dimension "d43" = 14.478
  dimension "d44" = 14.478
  dimension "d45" = 14.478
  dimension "d46" = 14.478
  dimension "d47" = 14.478
  dimension "d48" = 14.478
  dimension "d49" = 14.478
  dimension "d50" = 14.478
  dimension "d51" = 14.478
  dimension "d52" = 14.478
  dimension "d53" = 14.478
  dimension "d54" = 14.478
  dimension "d55" = 14.478
  dimension "d56" = 7.239
  dimension "d57" = 14.478
  dimension "d58" = 14.478
  dimension "d59" = 7.239
  dimension "d60" = 14.478
  dimension "d61" = 14.478
  dimension "d62" = 14.478
  dimension "d63" = 14.478
  dimension "d64" = 14.478
  dimension "d65" = 14.478
  constraints: 418 end point, 63 parallel, 57 midpoint, 35 horizontal, 35 perpendicular, 4 vertical, 3 point on line
  measures "d2" distance of L27.end L26.end
  measures "d3" distance of L26.end L25.end
  measures "d4" distance of L34.end L35.end
  measures "d5" distance of L33.end L34.end
  measures "d6" distance of L41.end L40.end
  measures "d7" distance of L40.end L39.end
  measures "d8" distance of L47.end L46.end
  measures "d9" distance of L46.end L45.end
  measures "d10" distance of L53.end L52.end
  measures "d11" distance of L52.end L51.end
  measures "d12" distance of L59.end L58.end
  measures "d13" distance of L58.end L57.end
  measures "d14" distance of L65.end L64.end
  measures "d15" distance of L64.end L63.end
  measures "d16" distance of L71.end L70.end
  measures "d17" distance of L69.end L70.end
  measures "d18" distance of L77.end L76.end
  measures "d19" distance of L76.end L75.end
  measures "d20" distance of L83.end L82.end
  measures "d21" distance of L82.end L81.end
  measures "d22" distance of L89.end L88.end
  measures "d23" distance of L88.end L87.end
  measures "d24" distance of L95.end L94.end
  measures "d25" distance of L94.end L93.end
  measures "d26" distance of L101.end L100.end
  measures "d27" distance of L100.end L99.end
  measures "d28" distance of L107.end L106.end
  measures "d29" distance of L106.end L105.end
  measures "d30" distance of L113.end L112.end
  measures "d31" distance of L112.end L111.end
  measures "d32" distance of L119.end L118.end
  measures "d33" distance of L118.end L117.end
  measures "d34" distance of L125.end L124.end
  measures "d35" distance of L124.end L123.end
  measures "d36" distance of L131.end L130.end
  measures "d37" distance of L130.end L129.end
  measures "d38" distance of L137.end L136.end
  measures "d39" distance of L136.end L135.end
  measures "d40" distance of L143.end L142.end
  measures "d41" distance of L142.end L141.end
  measures "d42" distance of L149.end L148.end
  measures "d43" distance of L148.end L147.end
  measures "d44" distance of L155.end L154.end
  measures "d45" distance of L154.end L153.end
  measures "d46" distance of L161.end L160.end
  measures "d47" distance of L160.end L159.end
  measures "d48" distance of L167.end L166.end
  measures "d49" distance of L166.end L165.end
  measures "d50" distance of L173.end L172.end
  measures "d51" distance of L172.end L171.end
  measures "d52" distance of L179.end L178.end
  measures "d53" distance of L178.end L177.end
  measures "d54" distance of L185.end L184.end
  measures "d55" distance of L184.end L183.end
  measures "d56" distance from line of L194 point (193.082, -146.168)
  measures "d57" distance of L191.start L191.end
  measures "d58" distance of L191.end L192.end
  measures "d59" distance from line of L193 L190.start
  measures "d60" distance of L198.end L195.end
  measures "d61" distance of L195.end L196.end
  measures "d62" distance of L202.end L199.end
  measures "d63" distance of L199.end L200.end
  measures "d64" distance of L206.end L203.end
  measures "d65" distance of L203.end L204.end
extrude "Extrusion1" add sketch "Sketch1" along normal blind 1.5875 contours L8 L232 L233 L231 A8 L7 A7 L6 A6 L5 A5 L4 A4 L3 A3 L2 A2 L1 A1 L0 A0 | L137 A20 | L143 A23 | L185 A31 | L179 A38 | L173 A40 | L149 A44 | L155 A51 | L161 A54 | L194 A60 | L202 A68 | L198 A73 | L167 A83 | A90 | A92 L214 L217 | A92 L217 A94 L210 L207 L208 L209 L214 | L217 A94 | A93 | A95 | A96 | A97 | A98 L206 | A98 L206 L203 L204 L205 | L206 A98 | L131 A110 | L125 A114 | L65 A122 | L71 A127 | L119 A132 | L107 A142 | L113 A146 | L27 A163 | L33 A165 | L77 A167 | L83 A173 | L89 A175 | L41 A178 | L53 A186 | L47 A187 | L101 A193 | L95 A232 | A241 | A242 | A244 | L59 A247 | A252 | A256 | A257 | A260 | A262 picked at (91.7683, -119.7564) picked at (109.7683, -119.7564) picked at (127.5564, -131.7335) picked at (145.7683, -129.2564) picked at (163.7683, -131.7564) picked at (127.6636, -114.7335) picked at (145.6636, -112.2335) picked at (163.6636, -114.7335) picked at (195.4249, -139.2697) picked at (233.4824, -153.1215) picked at (214.4536, -146.1956) picked at (181.6636, -117.2335) picked at (211.9939, -132.6345) picked at (213.8688, -128.8041) picked at (91.7683, -102.7564) picked at (109.7683, -102.7564) picked at (91.7683, -85.7564) picked at (109.7683, -85.7564) picked at (127.6636, -97.7335) picked at (163.6636, -97.7335) picked at (145.6636, -95.2335) picked at (91.7683, -68.7564) picked at (109.7683, -68.7564) picked at (127.6636, -80.7335) picked at (145.6636, -78.2335) picked at (163.6636, -80.7335) picked at (127.7683, -63.7564) picked at (163.7683, -63.7564) picked at (145.7683, -61.2564) picked at (181.6636, -100.2335) picked at (181.6636, -83.2335) picked at (181.6636, -66.2335)
fillet "Fillet1" radius 1.5875 4 edges at (218.4558, -105.5669, 0.7937) (204.8683, -105.5669, 0.7937) (218.4679, -95.4919, 0.7937) (204.8683, -95.4919, 0.7937)
equation "\"d3\" = d2"
body "Solid1"
